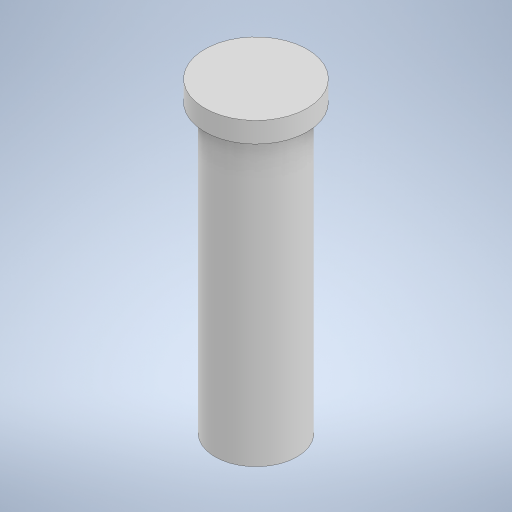
# Autodesk Inventor part: Shaft
Saved by Autodesk Inventor 2023 (Build 270158000, 158)
## iProperties
Created: 2023-02-02
Part Number: Shaft
Material: Generic
Document SubType Name: Modeling
Designer: MOHIKA
Density: 1 g/cm^3
Appearance: Default
Author: MOHIKA
Autodesk Inventor part; units mm, degrees
ref_plane "YZ Plane" through (0, 0, 0) normal (1, 0, 0) x (0, 1, 0)
ref_plane "XZ Plane" through (0, 0, 0) normal (0, 1, 0) x (-1, 0, 0)
ref_plane "XY Plane" through (0, 0, 0) normal (0, 0, 1) x (1, 0, 0)
sketch "Sketch1" plane through (0, 0, 0) normal (0, 0, 1) x (1, 0, 0)
  line L0 (0, 0) -> (0, 30)
  line L1 (0, 30) -> (5, 30)
  line L2 (5, 30) -> (5, 28)
  line L3 (5, 28) -> (4, 28)
  line L4 (4, 28) -> (4, 0)
  line L5 (4, 0) -> (0, 0)
  dimension "d0" = 30
  dimension "d1" = 5
  dimension "d2" = 2
  dimension "d3" = 1
  dimension "d4" = 28
  dimension "d5" = 4
  constraints: 12 end point, 2 perpendicular, 1 horizontal, 1 parallel, 1 vertical
  measures "d0" distance of L0.start L0.end
  measures "d1" distance of L0.end L1.end
  measures "d2" distance of L1.end L2.end
  measures "d3" distance of L2.end L3.end
  measures "d4" distance of L3.end L4.end
  measures "d5" distance of L4.end L0.start
revolve "Revolution1" add sketch "Sketch1" angle 360 about axis through (0, 0, 0) along (0, 1, 0)
body "Solid1"
